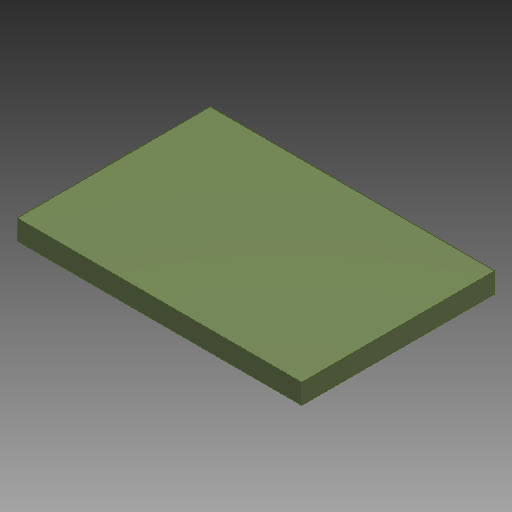
# Autodesk Inventor part: J1_SPC4077
Saved by Autodesk Inventor 2017.3 (Build 213256000, 256)
## iProperties
Part Number: J1_SPC4077
Material: Generisch
Document SubType Name: Modeling
Designer: Nils
Density: 1 g/cm^3
Appearance: SPC4077, J1_SPC4077
Author: Nils
Autodesk Inventor part; units mm, degrees
ref_plane "YZ Plane" through (0, 0, 0) normal (1, 0, 0) x (0, 1, 0)
ref_plane "XZ Plane" through (0, 0, 0) normal (0, 1, 0) x (-1, 0, 0)
ref_plane "XY Plane" through (0, 0, 0) normal (0, 0, 1) x (1, 0, 0)
sketch "SPC4077, J1_SPC4077_24" plane through (0, 0, 0) normal (0, 0, 1) x (1, 0, 0)
  line L0 (-10.8, 4.5) -> (3.5, 4.5)
  line L1 (3.5, 4.5) -> (3.5, -5.2)
  line L2 (3.5, -5.2) -> (-10.8, -5.2)
  line L3 (-10.8, -5.2) -> (-10.8, 4.5)
  constraints: 8 end point
extrude "Extrusion1" add sketch "SPC4077, J1_SPC4077_24" along normal blind 1
